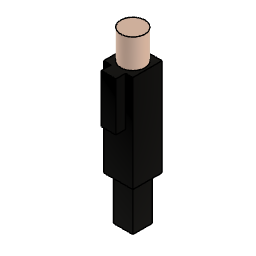
哈哈哈1 v8 v4 (Autodesk Fusion 360 design; units mm, degrees)
Autodesk Fusion 360 part; units mm, degrees
sketch "草图1" plane through (0, 0, 0) normal (0, 0, 1) x (1, 0, 0)
  line L0 (0, 0) -> (6, 0)
  line L1 (6, 0) -> (6, 6)
  line L2 (6, 6) -> (0, 6)
  line L3 (0, 6) -> (0, 0)
  constraint horizontal L0
  constraint vertical L1
  constraint horizontal L2
  constraint vertical L3
  constraint coincident L0.start L3.end
extrude "拉伸1" add sketch "草图1" along normal blind 20
sketch "草图2" plane through (0, 0, 0) normal (0, -1, 0) x (1, 0, 0)
  line L0 (0, 0) -> (6, 0)
  line L1 (6, 0) -> (6, 20)
  line L2 (6, 20) -> (0, 20)
  line L3 (0, 20) -> (0, 0)
  line L4 (0, 20) -> (1.5, 20)
  line L5 (1.5, 20) -> (1.5, 10)
  line L6 (1.5, 10) -> (0, 10)
  line L7 (0, 10) -> (0, 20)
  line L8 (0, 10) -> (0, 20)
  line L9 (0, 20) -> (1.5, 20)
  line L10 (1.5, 20) -> (1.5, 10)
  line L11 (0, 10) -> (0, 20)
  line L12 (1.5, 10) -> (0, 10)
  line L13 (0, 10) -> (0, 20)
  line L14 (0, 10) -> (0, 20)
  line L15 (1.5, 20) -> (1.5, 10)
  line L16 (0, 10) -> (0, 20)
  line L17 (0, 20) -> (1.5, 20)
  line L18 (1.5, 20) -> (1.5, 10)
  line L19 (1.5, 10) -> (0, 10)
  line L20 (0, 10) -> (0, 20)
  line L21 (1.5, 10) -> (0, 10)
  line L22 (0, 20) -> (1.5, 20)
  line L23 (0, 10) -> (0, 20)
  line L24 (4.4997, 10.0138) -> (4.4997, 20.0138)
  line L25 (5.9997, 20.0138) -> (5.9997, 10.0138)
  line L26 (4.4997, 10.0138) -> (4.4997, 20.0138)
  line L27 (4.4997, 20.0138) -> (5.9997, 20.0138)
  line L28 (5.9997, 20.0007) -> (5.9997, 10.0007)
  line L29 (5.9997, 10.0138) -> (4.4997, 10.0138)
  line L30 (4.4997, 10.0007) -> (4.4997, 20.0007)
  line L31 (5.9997, 10.0007) -> (4.4997, 10.0007)
  line L32 (4.4997, 20.0007) -> (5.9997, 20.0007)
  line L33 (4.4997, 10.0138) -> (4.4997, 20.0138)
  line L34 (1.5, 20) -> (4.4997, 20)
  line L35 (4.4997, 20) -> (4.4997, 10)
  line L36 (4.4997, 10) -> (1.5, 10)
  line L37 (1.5, 10) -> (1.5, 20)
  point P0 (0, 20)
  point P1 (0, 20)
  point P2 (0, 20)
  point P3 (4.4997, 20.0138)
  point P4 (4.4997, 20.0007)
  dimension "d3" = 10
  dimension "d4" = 10
  dimension "d5" = 10
  dimension "d6" = 10
  dimension "d7" = 10
  dimension "d8" = 10
  dimension "d9" = 10
  dimension "d10" = 10
  dimension "d11" = 10
  dimension "d12" = 10
  dimension "d13" = 10
  dimension "d14" = 10
  dimension "d15" = 10
  constraint horizontal L4
  constraint vertical L5
  constraint horizontal L6
  constraint vertical L7
  constraint coincident P2 P1
  constraint vertical L8
  constraint horizontal L9
  constraint vertical L10
  constraint horizontal L12
  constraint vertical L13
  constraint vertical L11
  constraint horizontal L17
  constraint vertical L15
  constraint horizontal L19
  constraint vertical L16
  constraint vertical L14
  constraint horizontal L22
  constraint vertical L18
  constraint horizontal L21
  constraint vertical L20
  constraint vertical L23
  constraint horizontal L27
  constraint vertical L25
  constraint horizontal L29
  constraint vertical L26
  constraint coincident P3 L24.end
  constraint vertical L24
  constraint horizontal L32
  constraint vertical L28
  constraint horizontal L31
  constraint vertical L30
  constraint coincident P4 L30.end
  constraint vertical L33
  constraint horizontal L34
  constraint vertical L35
  constraint horizontal L36
  constraint vertical L37
  constraint coincident L24 L35.end
  measures "d3" distance of P2 L6.end
  measures "d4" distance of L6.end P2
  measures "d5" distance of L6.end P2
  measures "d6" distance of P2 L6.end
  measures "d7" distance of L6.end P2
  measures "d8" distance of P2 L6.end
  measures "d9" distance of P2 L6.end
  measures "d10" distance of L6.end P2
  measures "d11" distance of L24.start P3
  measures "d12" distance of P3 L24.start
  measures "d13" distance of P4 L30.start
  measures "d14" distance of L24.start P3
  measures "d15" distance of L4.end L5.end
extrude "拉伸2" add sketch "草图2" along normal blind 2 contours L2 L5 L10 L15 L18 L24 L26 L30 L33 L34 L35 L36 L37
sketch "草图3" plane through (0, 0, 20) normal (0, 0, 1) x (-1, 0, 0)
  line L0 (0, -6) -> (0, 0)
  line L1 (0, 0) -> (-1.5, 0)
  line L2 (-1.5, 0) -> (-1.5, 2)
  line L3 (-1.5, 2) -> (-4.4997, 2)
  line L4 (-4.4997, 2) -> (-4.4997, 0)
  line L5 (-4.4997, 0) -> (-6, 0)
  line L6 (-6, 0) -> (-6, -6)
  line L7 (-6, -6) -> (0, -6)
  circle A0 centre (-3, -3) radius 2.5
  dimension "d18" = 5
  measures "d18" diameter of A0
extrude "拉伸3" add sketch "草图3" along normal blind 6 contours A0
sketch "草图4" plane through (0, 0, 0) normal (0, 0, -1) x (1, 0, 0)
  line L0 (0, 0) -> (0, -6)
  line L1 (0, -6) -> (6, -6)
  line L2 (6, -6) -> (6, 0)
  line L3 (6, 0) -> (0, 0)
  line L4 (0, 0) -> (1, 0)
  line L5 (1, 0) -> (1, -6)
  line L6 (1, -6) -> (0, -6)
  line L7 (0, -6) -> (0, 0)
  line L8 (5, 0) -> (6, 0)
  line L9 (6, 0) -> (6, -6)
  line L10 (6, -6) -> (5, -6)
  line L11 (5, -6) -> (5, 0)
  line L12 (6, -5) -> (0, -5)
  line L13 (0, -5) -> (0, -6)
  line L14 (0, -6) -> (6, -6)
  line L15 (6, -6) -> (6, -5)
  line L16 (0, 0) -> (6, 0)
  line L17 (6, 0) -> (6, -1)
  line L18 (6, -1) -> (0, -1)
  line L19 (0, -1) -> (0, 0)
  line L20 (1, -1) -> (5, -1)
  line L21 (5, -1) -> (5, -5)
  line L22 (5, -5) -> (1, -5)
  line L23 (1, -5) -> (1, -1)
  constraint horizontal L4
  constraint vertical L5
  constraint horizontal L6
  constraint vertical L7
  constraint coincident L1 L5.end
  constraint coincident L0.start L3.end
  constraint horizontal L8
  constraint vertical L9
  constraint horizontal L10
  constraint vertical L11
  constraint coincident L1.end L2.start
  constraint coincident L3 L8.start
  constraint horizontal L12
  constraint vertical L13
  constraint horizontal L14
  constraint vertical L15
  constraint coincident L0.end L1.start
  constraint coincident L9 L12.start
  constraint horizontal L16
  constraint vertical L17
  constraint horizontal L18
  constraint vertical L19
  constraint coincident L9 L17.end
  constraint horizontal L20
  constraint vertical L21
  constraint horizontal L22
  constraint vertical L23
  constraint coincident L12 L21.end
  constraint coincident L11 L21.end
  constraint coincident L5 L20.start
  constraint coincident L18 L20.start
extrude "拉伸4" add sketch "草图4" along normal blind 6 contours L5 L11 L12 L18 L20 L21 L22 L23
sketch "草图5" plane through (0, 0, -6) normal (0, 0, -1) x (1, 0, 0)
  line L0 (5, -5) -> (5, -1)
  line L1 (5, -1) -> (1, -1)
  line L2 (1, -1) -> (1, -5)
  line L3 (1, -1) -> (5, -1)
  line L4 (5, -1) -> (5, -5)
  line L5 (1, -5) -> (1, -1)
  line L6 (1, -5) -> (2, -5)
  line L7 (2, -5) -> (2, -4.5)
  line L8 (2, -4.5) -> (4, -4.5)
  line L9 (4, -4.5) -> (4, -5)
  line L10 (4, -5) -> (5, -5)
  circle A0 centre (3, -3) radius 1
  dimension "d23" = 2
  constraint horizontal L3
  constraint vertical L4
  constraint vertical L5
  constraint coincident L0.start L4.end
  constraint coincident L1.end L2.start
  constraint coincident L2.end L5.start
  constraint perpendicular L5 L6
  constraint perpendicular L6 L7
  constraint perpendicular L7 L8
  constraint perpendicular L8 L9
  constraint perpendicular L4 L10
  measures "d23" diameter of A0
extrude "拉伸5" add sketch "草图5" along normal blind 3 contours L0 L1 L2 L3 L4 L5 L6 L7 L8 L9 L10 | A0
sketch "草图6" plane through (0, 0, -9) normal (0, 0, -1) x (1, 0, 0)
  line L0 (1, -5) -> (2, -5)
  line L1 (2, -5) -> (2, -4.5)
  line L2 (2, -4.5) -> (4, -4.5)
  line L3 (4, -4.5) -> (4, -5)
  line L4 (4, -5) -> (5, -5)
  line L5 (5, -5) -> (5, -1)
  line L6 (5, -1) -> (1, -1)
  line L7 (1, -1) -> (1, -5)
  circle A0 centre (3, -3) radius 1
  dimension "d26" = 2
  measures "d26" diameter of A0
extrude "拉伸6" cut sketch "草图6" against normal blind 1 contours A0
